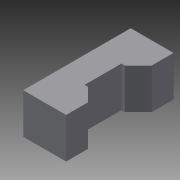
# Autodesk Inventor part: Limit Adapter
Saved by Autodesk Inventor 2015 (Build 190159000, 159)
## iProperties
Created: 2015-05-29
Part Number: Limit Adapter
Material: Generic
Document SubType Name: Modeling
Designer: pltwe4
Density: 1 g/cm^3
Appearance: Default
Author: pltwe4
Autodesk Inventor part; units mm, degrees
ref_plane "YZ Plane" through (0, 0, 0) normal (1, 0, 0) x (0, 1, 0)
ref_plane "XZ Plane" through (0, 0, 0) normal (0, 1, 0) x (-1, 0, 0)
ref_plane "XY Plane" through (0, 0, 0) normal (0, 0, 1) x (1, 0, 0)
sketch "Sketch1" plane through (0, 0, 0) normal (0, 0, 1) x (1, 0, 0)
  line L0 (-18.3846, 28.5) -> (-18.3846, 22)
  line L1 (-18.3846, 22) -> (-22.3846, 18)
  line L2 (-22.3846, 18) -> (-22.3846, 7)
  line L3 (-22.3846, 7) -> (-18.3846, 3)
  line L4 (-18.3846, 3) -> (-18.3846, -3.5)
  line L5 (-18.3846, 28.5) -> (-31.1346, 28.5)
  line L6 (-31.1346, 28.5) -> (-31.1346, -3.5)
  line L7 (-31.1346, -3.5) -> (-18.3846, -3.5)
  line L8 (-22.3846, 7) -> (-23.3846, 7)
  line L9 (-23.3846, 7) -> (-23.3846, 18)
  line L10 (-23.3846, 18) -> (-22.3846, 18)
  line L11 (-31.1346, 11.0301) -> (-37.4846, 11.0301) construction
  point P0 (0, 0)
  dimension "d0" = 1
  dimension "d1" = 6.35
  dimension "d2" = 8.75
  dimension "d13" = 135
  dimension "d14" = 135
  dimension "d15" = 11
  dimension "d16" = 12.75
  dimension "d17" = 32
  constraints: 24 end point, 6 perpendicular, 3 horizontal, 2 equal length, 1 point on line
  measures "d0" distance between parallel lines of L2 L9
  measures "d1" distance of L11.start L11.end
  measures "d2" distance between parallel lines of L2 L6
  measures "d13" angle of L0 L1
  measures "d14" angle of L4 L3
  measures "d15" distance of L1.end L2.end
  measures "d16" distance of L0.start L5.end
  measures "d17" distance of L5.end L6.end
extrude "Extrusion1" add sketch "Sketch1" against normal blind 12 contours L0 L1 L10 L9 L8 L3 L4 L7 L6 L5
sketch "Sketch3" plane through (-31.1346, -3.5, 0) normal (-1, 0, 0) x (0, 0, 1)
  line L0 (0, 32) -> (0, 0) projected
  line L1 (0, 32) -> (-12, 32) projected
  line L2 (-12, 0) -> (-12, 32) projected
  line L3 (0, 0) -> (-12, 0) projected
  circle A0 centre (-7.62, 11.25) radius 1.27
  circle A1 centre (-7.62, 20.75) radius 1.27
  line L4 (-12, 21.5) -> (-12, 10.5) construction
  line L5 (-12, 16) -> (0, 16) construction
  point P0 (0, 3.5)
  dimension "d8" = 2.54
  dimension "d9" = 9.5
  dimension "d10" = 7.62
  constraints: 2 centre point, 2 end point, 2 midpoint, 1 equal radius, 1 other
  measures "d8" diameter of A0
  measures "d9" distance of A1.centre A0.centre
  measures "d10" distance from line of A1.centre L0
extrude "Extrusion3" add sketch "Sketch3" along normal blind 5 contours A0 | A1
body "Solid1"
